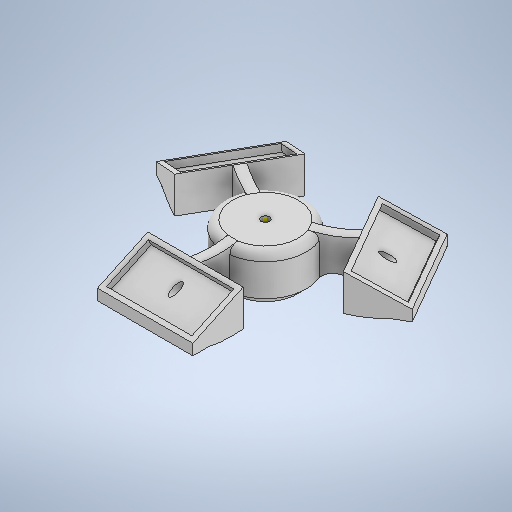
# Autodesk Inventor part: Water_Sensor_Cap
Saved by Autodesk Inventor 2025 (Build 290162000, 162)
## iProperties
Created: 2024-06-19
Part Number: Water_Sensor_Cap
Material: Generic
Document SubType Name: Modeling
Designer: track
Density: 1 g/cm^3
Appearance: Default
Mass: 56.6087 g
Surface Area: 245.5 cm^2
Volume: 56.6087 cm^3
Author: track
## iProperties of the stored document Water_Sensor_Cap_3DPrint.ipt
Created: 2024-06-19
Part Number: Water_Sensor_Cap_3DPrint
Material: Generic
Document SubType Name: Modeling
Designer: track
Density: 1 g/cm^3
Appearance: Default
Author: track
Autodesk Inventor part; units mm, degrees
ref_plane "YZ Plane" through (0, 0, 0) normal (1, 0, 0) x (0, 1, 0)
ref_plane "XZ Plane" through (0, 0, 0) normal (0, 1, 0) x (-1, 0, 0)
sketch "Sketch1" plane through (0, 0, 0) normal (0, 1, 0) x (-1, 0, 0)
  circle A0 centre (0, 0) radius 30.48
  circle A1 centre (0, 0) radius 32.48
  dimension "d0" = 60.96
  dimension "d2" = 2
  constraints: 2 centre point, 2 coincident
  measures "d0" diameter of A0
  measures "d2" radial gap between concentric circles of A1 A0
extrude "Extrusion1" add sketch "Sketch1" along normal blind 19.05
sketch "Sketch2" plane through (0, 19.05, 0) normal (0, 1, 0) x (1, 0, 0)
  circle A0 centre (0, 0) radius 32.48
  circle A1 centre (0, 0) radius 32.48 projected
  constraints: 1 centre point, 1 coincident, 1 concentric
extrude "Extrusion2" add sketch "Sketch2" along normal blind 12.7 and the other way blind 6.35
fillet "Fillet1" radius 6.35 1 edges at (-32.48, 31.75, 0)
sketch "Sketch3" plane through (0, 31.75, 0) normal (0, 1, 0) x (1, 0, 0)
  point P0 (0, 0)
sketch "Sketch6" plane through (0, 31.75, 0) normal (0, 1, 0) x (1, 0, 0)
  circle A0 centre (0, 0) radius 3.302
  dimension "d15" = 6.604
  constraints: 1 centre point, 1 coincident
  measures "d15" diameter of A0
extrude "Extrusion5" cut sketch "Sketch6" against normal up to surface (19.05 mm away)
sketch "Sketch9" plane through (0, 12.7, 0) normal (0, -1, 0) x (1, 0, 0)
  point P0 (0, 0)
sketch "Sketch10" plane through (0, 0, 0) normal (0, 0, 1) x (1, 0, 0)
  line L0 (-17.78, 19.05) -> (-17.78, -11.43)
  line L1 (-17.78, -11.43) -> (-25.4, -11.43)
  line L2 (-25.4, -11.43) -> (-25.4, 19.05)
  line L3 (-17.78, 19.05) -> (-25.4, 19.05)
  line L4 (-26.13, 31.75) -> (26.13, 31.75) projected
  line L5 (0, 31.75) -> (0, 0)
  line L6 (32.48, 0) -> (-32.48, 0) projected
  line L7 (-30.48, 0) -> (-30.48, 19.05)
  line L8 (-17.78, -11.43) -> (-25.4, -7.0306)
  line L9 (30.48, 12.7) -> (-30.48, 12.7) projected
  point P0 (-17.78, 12.7)
  point P1 (-25.4, 12.7)
  dimension "d29" = 7.62
  dimension "d33" = 30
  dimension "d42" = 25.4
  dimension "d89" = 24.13
  constraints: 14 end point, 4 perpendicular, 2 point on line, 2 vertical, 1 midpoint
  measures "d29" distance between parallel lines of L0 L2
  measures "d33" angle of L1 L8
  measures "d42" distance between parallel lines of L5 L2
  measures "d89" distance between parallel lines of L9 L1
revolve "Revolution2" add sketch "Sketch10" angle 360 about axis through (0, 31.75, 0) along (0, -1, 0) contours L0 L6 L2 L9 | L0 L8 L2 L6
sketch "Sketch11" plane through (0, 0, 0) normal (0, 0, 1) x (1, 0, 0)
  line L0 (25.4, -7.0306) -> (25.4, 25.4)
  circle A0 centre (26.3462, -2.54) radius 2.3813
  circle A1 centre (26.3461, 3.81) radius 2.3813
  line L1 (-25.4, -7.0306) -> (25.4, -7.0306) projected
  line L2 (0, -11.43) -> (0, 31.75)
  line L3 (-26.13, 31.75) -> (26.13, 31.75) projected
  line L4 (26.3461, 3.81) -> (26.3462, -2.54)
  line L5 (30.48, 12.7) -> (30.48, 0) projected
  line L6 (30.48, 0) -> (29.972, 19.05)
  line L7 (29.972, 12.7) -> (29.972, 0) projected
  line L8 (-25.4, -11.43) -> (25.4, -11.43) projected
  line L9 (-17.78, -11.43) -> (17.78, -11.43) projected
  point P0 (0, 0)
  point P1 (27.772, -0.6806)
  dimension "d36" = 6.35
  dimension "d37" = 4.7625
  dimension "d38" = 4.7625
  dimension "d43" = 26.3462
  dimension "d91" = 8.89
  constraints: 8 end point, 2 centre point, 2 vertical, 1 midpoint, 1 point on line, 3 other
  measures "d36" distance of L4.end L4.start
  measures "d37" diameter of A1
  measures "d38" diameter of A0
  measures "d43" distance between parallel lines of L2 L4
  measures "d91" distance from line of L9 L4.end
revolve "Revolution3" cut sketch "Sketch11" angle 360 about axis through (0, -11.43, 0) along (0, 1, 0) contours A0 L0 | L0 A0 | A1 L0 | L0 A1
ref_plane "Work Plane1" through (0, 0, 32.48) normal (0, 0, 1) x (1, 0, 0)
sketch "Sketch12" plane through (0, 0, 32.48) normal (0, 0, 1) x (1, 0, 0)
  line L0 (-4, 31.75) -> (4, 31.75)
  line L1 (4, 31.75) -> (4, -8.25)
  line L2 (4, -8.25) -> (-4, -8.25)
  line L3 (-4, -8.25) -> (-4, 31.75)
  line L4 (-4, 31.75) -> (4, -8.25) construction
  line L5 (4, 31.75) -> (-4, -8.25) construction
  line L6 (-26.13, 31.75) -> (26.13, 31.75) projected
  point P0 (0, 0)
  point P1 (0, 11.75)
  dimension "d44" = 40
  dimension "d45" = 0
  dimension "d46" = 8
  dimension "d47" = 0
  constraints: 12 end point, 2 midpoint, 2 parallel, 1 horizontal, 1 perpendicular
  measures "d44" distance of L0.end L1.end
  measures "d45" distance between parallel lines of L6 L0
  measures "d46" distance of L0.start L0.end
  measures "d47" horizontal distance of point (0, 11.75) point (0, 0)
extrude "Extrusion7" add sketch "Sketch12" along normal blind 23 and the other way blind 7
sketch "Sketch14" plane through (-4, -8.25, 55.48) normal (0, -1, 0) x (1, 0, 0)
  circle A0 centre (4, -55.48) radius 30.48
  circle A1 centre (4, -55.48) radius 25.4
  arc A2 (0, -25.2636) -> (8, -25.2636) centre (4, -55.48) ccw projected
  circle A3 centre (4, -55.48) radius 25.4 projected
  constraints: 2 centre point, 2 coincident, 2 concentric
extrude "Extrusion8" cut sketch "Sketch14" against normal up to surface (20.95 mm away)
sketch "Sketch15" plane through (4, -8.25, 55.48) normal (1, 0, 0) x (0, 0, -1)
  line L0 (23.2472, 33.65) -> (23.2472, 8.25) projected
  line L1 (23.2472, 8.25) -> (25.2636, 8.25) projected
  line L2 (23.2472, 8.25) -> (25.2636, 8.25)
  line L3 (25.2636, 8.25) -> (25.2636, 0)
  line L4 (25.2636, 0) -> (25, 0) projected
  line L5 (0, 40) -> (0, 0) projected
  line L6 (25.2636, 0) -> (0, 0)
  arc A0 (23.2472, 8.25) -> (0, 0) centre (13.0875, 0) ccw
  line L7 (0, 0) -> (0, 40) projected
  line L8 (29.658, 40) -> (81.61, 40) projected
  arc A1 (0, 40) -> (29.658, 40) centre (14.829, 114.7432) ccw
  line L9 (29.658, 40) -> (0, 40) projected
  line L10 (0, 40) -> (29.658, 40)
  point P0 (55.48, 8.25)
  dimension "d54" = 76.2
  constraints: 8 end point, 4 point on circle, 2 centre point, 2 collinear, 2 perpendicular, 1 tangent
  measures "d54" radius of A1
extrude "Extrusion9" cut sketch "Sketch15" against normal up to surface (8 mm away)
sketch "Sketch17" plane through (4, -8.25, 55.48) normal (1, 0, 0) x (0, 0, -1)
  line L0 (0, 40) -> (0, 0) projected
  line L1 (0, 40) -> (-40, 21.3477)
  line L2 (-40, 21.3477) -> (-40, 0)
  line L3 (-40, 0) -> (0, 0)
  point P0 (55.48, 8.25)
  dimension "d61" = 40
  dimension "d63" = 115
  constraints: 6 end point, 1 parallel, 1 perpendicular
  measures "d61" distance between parallel lines of L0 L2
  measures "d63" angle of L2 L1
extrude "Extrusion10" add sketch "Sketch17" along normal blind 33.875 and the other way blind 41.875
sketch "Sketch18" plane through (-37.875, 13.0977, 95.48) normal (0, 0.9063078, 0.4226183) x (1, 0, 0)
  line L0 (71.75, 3.5751) -> (4, 3.5751)
  line L1 (4, 3.5751) -> (4, 40.3251)
  line L2 (4, 40.3251) -> (71.75, 40.3251)
  line L3 (71.75, 40.3251) -> (71.75, 3.5751)
  line L4 (71.75, 3.5751) -> (4, 40.3251) construction
  line L5 (4, 3.5751) -> (71.75, 40.3251) construction
  ellipse E0 centre (37.875, 86.3662) end of major axis (41.177, 86.3662) minor radius 2.9926 projected
  line L6 (41.875, 44.1351) -> (75.75, 44.1351) projected
  point P0 (37.875, 80.9989)
  point P1 (37.875, 21.9501)
  dimension "d68" = 67.75
  dimension "d69" = 36.75
  dimension "d70" = 0
  dimension "d71" = 3.81
  constraints: 12 end point, 2 midpoint, 2 parallel, 1 horizontal, 1 perpendicular
  measures "d68" distance of L1.end L2.end
  measures "d69" distance of L0.end L1.end
  measures "d70" horizontal distance of E0.centre point (37.875, 21.95)
  measures "d71" distance between parallel lines of L6 L2
extrude "Extrusion11" cut sketch "Sketch18" against normal blind 5 contours L0 L1 L2 L3
sketch "Sketch19" plane through (37.875, -8.25, 55.48) normal (1, 0, 0) x (0, 0, -1)
  line L0 (-40, 0) -> (-40, 21.3477) projected
  line L1 (-40, 12.7) -> (-27.6329, 12.7)
  arc A0 (23.2472, 8.25) -> (0, 0) centre (13.0875, 0) ccw projected
  line L2 (-40, 0) -> (0, 0) projected
  line L3 (0, 40) -> (-40, 21.3477) projected
  line L4 (-40, 12.7) -> (-40, 0)
  arc A1 (-26.98, 12.6322) -> (10.2914, 12.7853) centre (-8.7015, 99.6328) ccw
  arc A2 (-26.98, 12.6322) -> (-27.6329, 12.7) centre (-27.6329, 9.525) ccw
  arc A3 (10.2914, 12.7853) -> (0, 0) centre (13.0875, 0) ccw
  point P0 (55.48, 8.25)
  point P1 (-27.3, 12.7)
  dimension "d75" = 12.7
  dimension "d84" = 88.9
  dimension "d85" = 12.7
  dimension "d86" = 3.175
  constraints: 8 point on circle, 4 end point, 4 tangent, 3 centre point, 2 point on line, 1 collinear, 1 horizontal
  measures "d75" distance between parallel lines of L2 L1
  measures "d84" radius of A1
  measures "d85" distance of L1.start point (-27.3, 12.7)
  measures "d86" radius of A2
extrude "Extrusion12" cut sketch "Sketch19" against normal up to surface (75.75 mm away)
ref_plane "Work Plane3" through (0, 0, 80.9625) normal (0, 0, 1) x (1, 0, 0)
sketch "Sketch21" plane through (0, 0, 80.9625) normal (0, 0, 1) x (1, 0, 0)
  circle A0 centre (0, 18.9671) radius 2.5
  line L0 (33.875, 10.0771) -> (-33.875, 10.0771) projected
  line L1 (33.875, 30.1398) -> (33.875, 14.6086) projected
  point P0 (0, 0)
  dimension "d93" = 5
  dimension "d94" = 8.89
  dimension "d95" = 33.875
  constraints: 1 centre point
  measures "d93" diameter of A0
  measures "d94" distance from line of L0 A0.centre
  measures "d95" distance from line of L1 A0.centre
extrude "Extrusion13" cut sketch "Sketch21" against normal blind 71.4375
sketch "Sketch22" plane through (0, 12.7, 0) normal (0, -1, 0) x (1, 0, 0)
  circle A0 centre (0, 0) radius 3.302 projected
  circle A1 centre (0, 0) radius 17.78
  circle A2 centre (0, 0) radius 17.78 projected
  constraints: 1 centre point, 1 coincident, 1 concentric
extrude "Extrusion14" cut sketch "Sketch22" against normal blind 12.7
pattern_circular "Circular Pattern3" count 3 over 360 about axis through (0, 25.4, 0) along (0, 1, 0) of "Extrusion13", "Extrusion12", "Extrusion11", "Extrusion10", "Extrusion9", "Extrusion8", "Extrusion7"
body "Solid1"
